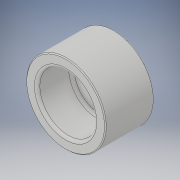
# Autodesk Inventor part: Диана деталь
Saved by Autodesk Inventor 2019.3 (Build 233278000, 278)
## iProperties
Created: 2020-03-24
Part Number: Диана деталь
Material: Типовые
Document SubType Name: Modeling
Designer: Admin
Density: 1 g/cm^3
Appearance: По умолчанию
Author: Admin
Autodesk Inventor part; units mm, degrees
ref_plane "YZ Plane" through (0, 0, 0) normal (1, 0, 0) x (0, 1, 0)
ref_plane "XZ Plane" through (0, 0, 0) normal (0, 1, 0) x (-1, 0, 0)
ref_plane "XY Plane" through (0, 0, 0) normal (0, 0, 1) x (1, 0, 0)
sketch "Эскиз1" plane through (0, 0, 0) normal (0, 0, 1) x (1, 0, 0)
  circle A0 centre (0, 0) radius 22
  dimension "d0" = 44
  constraints: 1 centre point, 1 coincident
  measures "d0" diameter of A0
extrude "Выдавливание1" add sketch "Эскиз1" along normal blind 27
sketch "Эскиз2" plane through (0, 0, 27) normal (0, 0, 1) x (1, 0, 0)
  point P0 (0, 0)
  point P1 (0, 0)
  constraints: 1 coincident
hole "Отверстие1" at (0, 0, 27) direction (0, 0, -1) diameter 31.5 depth 19
sketch "Эскиз3" plane through (0, 0, 0) normal (0, 0, -1) x (-1, 0, 0)
  point P0 (0, 0)
  point P1 (0, 0)
  constraints: 1 coincident
hole "Отверстие2" at (0, 0, 0) direction (0, 0, 1) diameter 5.917 end through all thread size "M7x1" class "6H" standard "ANSI Metric M Profile"
fillet "Сопряжение1" radius 0.5 1 edges at (-22, 0, 0)
chamfer "Фаска1" distance 0.5 angle 45 1 edges at (-22, 0, 27)
fillet "Сопряжение2" radius 1.5 2 edges at (0, 15.75, 27) (0, 15.75, 8)
chamfer "Фаска2" distance 0.25 angle 45 1 edges at (0, -2.9585, 8)
